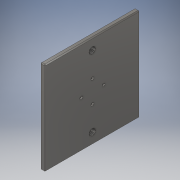
# Autodesk Inventor part: plytkaadaptacyjna
Saved by Autodesk Inventor 2019 (Build 230136000, 136)
## iProperties
Created: 2020-08-30
Part Number: plytkaadaptacyjna
Material: Stainless Steel
Document SubType Name: Modeling
Designer: estee
Density: 8 g/cm^3
Appearance: Semi-Polished
Author: estee
Autodesk Inventor part; units mm, degrees
ref_plane "YZ Plane" through (0, 0, 0) normal (1, 0, 0) x (0, 1, 0)
ref_plane "XZ Plane" through (0, 0, 0) normal (0, 1, 0) x (-1, 0, 0)
ref_plane "XY Plane" through (0, 0, 0) normal (0, 0, 1) x (1, 0, 0)
sketch "Sketch1" plane through (0, 0, 0) normal (1, 0, 0) x (0, 1, 0)
  point P0 (0, 0)
  point P1 (0, 12)
  dimension "d0" = 12
  measures "d0" distance of point (0, 0) point (0, 12)
sketch "Sketch2" plane through (0, 0, 0) normal (1, 0, 0) x (0, 1, 0)
  line L0 (-50, 51) -> (50, 51)
  line L1 (50, 51) -> (50, -51)
  line L2 (50, -51) -> (-50, -51)
  line L3 (-50, -51) -> (-50, 51)
  line L4 (-50, 51) -> (50, -51) construction
  line L5 (50, 51) -> (-50, -51) construction
  point P0 (0, 0)
  dimension "d1" = 100
  dimension "d2" = 102
  constraints: 12 end point, 2 midpoint, 2 parallel, 1 horizontal, 1 perpendicular
  measures "d1" distance of L1.end L2.end
  measures "d2" distance of L0.end L1.end
extrude "Extrusion1" add sketch "Sketch2" along normal blind 5
hole "Hole1" at (0, 0, 12) direction (1, 0, 0) diameter 3.2 end through all counterbore diameter 6 counterbore depth 3.4
pattern_circular "Circular Pattern1" count 4 over 360 about axis through (-10, 0, 0) along (1, 0, 0) of "Hole1"
sketch "Sketch3" plane through (0, 0, 0) normal (-1, 0, 0) x (0, 0, 1)
  point P0 (0, 0)
  point P1 (0, 38.1)
  point P2 (0, -38.1)
  dimension "d15" = 38.1
  dimension "d16" = 38.1
  measures "d15" distance of point (0, 0) point (0, 38.1)
  measures "d16" distance of point (0, 0) point (0, -38.1)
hole "Hole2" at (0, -38.1, 0) at (0, 38.1, 0) direction (1, 0, 0) diameter 6.647 end through all thread size "M8x1.25" class "6H" standard "ISO Metric profile"
chamfer "Chamfer1" distance 1 angle 45 12 edges at (0, 0, -51) (0, -50, 0) (0, 0, 51) (0, 50, 0) (2.5, 50, 51) (5, 0, 51) (2.5, -50, 51) (5, -50, 0) (2.5, -50, -51) (5, 0, -51) (2.5, 50, -51) (5, 50, 0)
chamfer "Chamfer2" distance 0.3 angle 45 8 edges at (0, 0, 9) (0, -9, 0) (0, 9, 0) (0, 0, -9) (0, -38.1, -3.3235) (0, 38.1, -3.3235) (5, -38.1, -3.3235) (5, 38.1, -3.3235)
body "Solid1"
